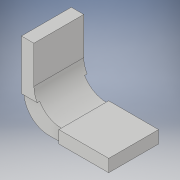
# Autodesk Inventor part: elbow
Saved by Autodesk Inventor 2017 (Build 210142000, 142)
## iProperties
Created: 2016-12-07
Part Number: elbow
Material: Generic
Document SubType Name: Modeling
Designer: PLTW
Density: 1 g/cm^3
Appearance: Default
Author: PLTW
Autodesk Inventor part; units mm, degrees
ref_plane "YZ Plane" through (0, 0, 0) normal (1, 0, 0) x (0, 1, 0)
ref_plane "XZ Plane" through (0, 0, 0) normal (0, 1, 0) x (-1, 0, 0)
ref_plane "XY Plane" through (0, 0, 0) normal (0, 0, 1) x (1, 0, 0)
sketch "Sketch1" plane through (0, 0, 0) normal (0, 1, 0) x (-1, 0, 0)
  line L0 (-3.175, -3.175) -> (3.175, -3.175)
  line L1 (3.175, -3.175) -> (3.175, 3.175)
  line L2 (3.175, 3.175) -> (-3.175, 3.175)
  line L3 (-3.175, 3.175) -> (-3.175, -3.175)
  line L4 (-3.175, -3.175) -> (3.175, 3.175) construction
  line L5 (3.175, -3.175) -> (-3.175, 3.175) construction
  line L6 (6.35, -2.8575) -> (3.175, -2.8575)
  line L7 (3.175, -2.8575) -> (3.175, 2.8575)
  line L8 (3.175, 2.8575) -> (6.35, 2.8575)
  line L9 (6.35, 2.8575) -> (6.35, -2.8575)
  line L10 (6.35, -2.8575) -> (3.175, 2.8575) construction
  line L11 (3.175, -2.8575) -> (6.35, 2.8575) construction
  point P0 (0, 0)
  point P1 (4.7625, 0)
  point P2 (4.7625, 0)
  point P3 (0, 0)
  dimension "d0" = 6.35
  dimension "d1" = 3.175
  dimension "d2" = 5.715
  constraints: 24 end point, 6 midpoint, 4 parallel, 3 perpendicular, 2 horizontal, 1 horizontal alignment, 1 point on line
  measures "d0" distance of L0.start L0.end
  measures "d1" distance of L7.end L8.end
  measures "d2" distance of L8.end L6.start
extrude "Extrusion1" add sketch "Sketch1" along normal blind 1.5875
pattern_circular "Circular Pattern1" count 2 over 90 about axis through (-6.35, 0, -2.8575) along (0, 0, 1) of "Extrusion1"
fillet "Fillet1" radius 3.175 2 edges at (-6.35, 1.5875, 0) (-7.9375, 0, 0)
body "Solid1"
